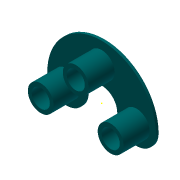
# Autodesk Inventor part: Island
Saved by Autodesk Inventor 2015 (Build 190159000, 159)
## iProperties
Created: 2015-03-07
Part Number: Island
Material: Generic
Document SubType Name: Modeling
Designer: Vukica
Density: 1 g/cm^3
Appearance: Default
Author: Vukica
Autodesk Inventor part; units mm, degrees
ref_plane "YZ Plane" through (0, 0, 0) normal (1, 0, 0) x (0, 1, 0)
ref_plane "XZ Plane" through (0, 0, 0) normal (0, 1, 0) x (-1, 0, 0)
ref_plane "XY Plane" through (0, 0, 0) normal (0, 0, 1) x (1, 0, 0)
sketch "Sketch1" plane through (0, 0, 0) normal (0, 0, 1) x (1, 0, 0)
  arc A0 (342.9, 0) -> (-342.9, 0) centre (0, 0) ccw construction
  arc A1 (533.4, 0) -> (-533.4, 0) centre (0, 0) ccw
  arc A2 (152.4, 0) -> (-152.4, 0) centre (0, 0) ccw
  arc A3 (152.4, 0) -> (533.4, 0) centre (342.9, 0) ccw
  arc A4 (-533.4, 0) -> (-152.4, 0) centre (-342.9, 0) ccw
  dimension "d0" = 152.4
  dimension "d1" = 381
  constraints: 10 point on circle, 5 centre point, 4 tangent, 1 coincident
  measures "d0" radius of A2
  measures "d1" radial gap between concentric circles of A2 A1
extrude "Extrusion1" add sketch "Sketch1" along normal blind 25.4
sketch "Sketch2" plane through (0, 0, 25.4) normal (0, 0, 1) x (1, 0, 0)
  point P0 (0, 0)
sketch "Sketch3" plane through (0, 0, 25.4) normal (0, 0, 1) x (1, 0, 0)
  circle A0 centre (-342.9, 0) radius 190.5
  circle A1 centre (342.9, 0) radius 190.5
  arc A2 (-533.4, 0) -> (-152.4, 0) centre (-342.9, 0) ccw projected
  arc A3 (152.4, 0) -> (533.4, 0) centre (342.9, 0) ccw projected
  circle A4 centre (0, 342.9) radius 190.5
  arc A5 (533.4, 0) -> (-533.4, 0) centre (0, 0) ccw projected
  dimension "d4" = 381
  dimension "d5" = 381
  constraints: 3 centre point, 2 concentric, 1 equal radius, 1 tangent
  measures "d4" diameter of A0
  measures "d5" diameter of A4
extrude "Extrusion2" add sketch "Sketch3" along normal blind 152.4
sketch "Sketch4" plane through (0, 342.9, 177.8) normal (0, 0, 1) x (1, 0, 0)
  circle A0 centre (0, 0) radius 190.5 projected
  circle A1 centre (-342.9, -342.9) radius 190.5 projected
  circle A2 centre (342.9, -342.9) radius 190.5 projected
  circle A3 centre (0, 0) radius 165.1
  circle A4 centre (342.9, -342.9) radius 165.1
  circle A5 centre (-342.9, -342.9) radius 165.1
  point P0 (0, -342.9)
  dimension "d35" = 330.2
  constraints: 3 centre point, 2 equal radius
  measures "d35" diameter of A3
extrude "Extrusion3" cut sketch "Sketch4" against normal blind 101.6 contours A3 | A4 | A5
equation "\"d5\" = d4"
body "Solid1"
